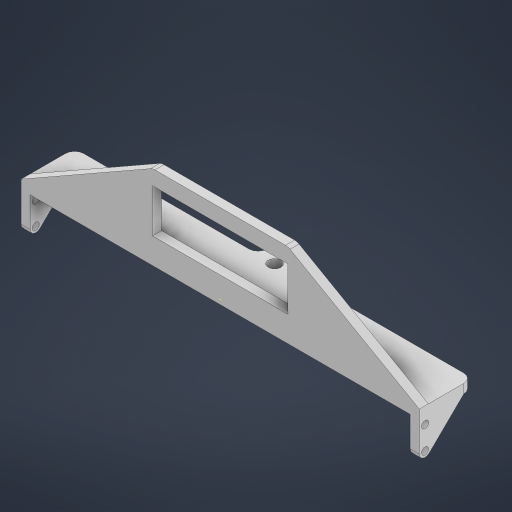
# Autodesk Inventor part: CS_Camera_Mount
Saved by Autodesk Inventor 2023 (Build 270158000, 158)
## iProperties
Created: 2024-02-10
Part Number: CS_Camera_Mount
Material: Generic
Document SubType Name: Modeling
Designer: kelle
Density: 1 g/cm^3
Appearance: Default
Author: kelle
Autodesk Inventor part; units mm, degrees
ref_plane "YZ Plane" through (0, 0, 0) normal (1, 0, 0) x (0, 1, 0)
ref_plane "XZ Plane" through (0, 0, 0) normal (0, 1, 0) x (-1, 0, 0)
ref_plane "XY Plane" through (0, 0, 0) normal (0, 0, 1) x (1, 0, 0)
sketch "Sketch1" plane through (0, 0, 0) normal (0, 0, 1) x (1, 0, 0)
  line L0 (139.7, -3.175) -> (-139.7, -3.175)
  line L1 (-139.7, -3.175) -> (-139.7, 3.175)
  line L2 (-139.7, 3.175) -> (139.7, 3.175)
  line L3 (139.7, 3.175) -> (139.7, -3.175)
  line L4 (139.7, -3.175) -> (-139.7, 3.175) construction
  line L5 (-139.7, -3.175) -> (139.7, 3.175) construction
  point P0 (0, 0)
  dimension "d0" = 279.4
  dimension "d1" = 6.35
  constraints: 12 end point, 2 midpoint, 2 parallel, 1 horizontal, 1 perpendicular
  measures "d0" distance of L1.end L2.end
  measures "d1" distance of L0.end L1.end
extrude "Extrusion1" add sketch "Sketch1" along normal blind 63.5
sketch "Sketch2" plane through (-139.7, 3.175, 0) normal (0, 1, 0) x (1, 0, 0)
  circle A0 centre (140.335, -26) radius 4.445
  line L0 (139.7, 0) -> (139.7, -63.5833) construction
  line L1 (0, 0) -> (0, -63.5) construction
  line L2 (279.4, 0) -> (279.4, -63.5) construction
  line L3 (279.4, -63.5) -> (0, -63.5) projected
  dimension "d4" = 8.89
  dimension "d16" = 37.5
  constraints: 2 end point, 1 centre point, 1 vertical
  measures "d4" diameter of A0
  measures "d16" distance from line of L3 A0.centre
extrude "Extrusion2" cut sketch "Sketch2" against normal through all
sketch "Sketch3" plane through (0, 0, 63.5) normal (0, 0, 1) x (1, 0, 0)
  point P0 (0, 0)
sketch "Sketch4" plane through (-139.7, 3.175, 0) normal (0, 1, 0) x (1, 0, 0)
  line L0 (279.4, 0) -> (279.4, -63.5) projected
  line L1 (0, 0) -> (0, -63.5) projected
  line L2 (279.4, -63.5) -> (0, -63.5)
  line L3 (0, -63.5) -> (0, -57.15)
  line L4 (0, -57.15) -> (279.4, -57.15)
  line L5 (279.4, -57.15) -> (279.4, -63.5)
  point P0 (139.7, 0)
  dimension "d8" = 6.35
  constraints: 8 end point, 2 parallel, 1 horizontal, 1 perpendicular, 1 point on line
  measures "d8" distance of L2.end L3.end
extrude "Extrusion3" add sketch "Sketch4" along normal blind 63.5
sketch "Sketch5" plane through (0, 0, 63.5) normal (0, 0, 1) x (1, 0, 0)
  line L0 (47.5, 14.825) -> (-47.5, 14.825)
  line L1 (-47.5, 14.825) -> (-47.5, 45.305)
  line L2 (-47.5, 45.305) -> (47.5, 45.305)
  line L3 (47.5, 45.305) -> (47.5, 14.825)
  line L4 (47.5, 14.825) -> (-47.5, 45.305) construction
  line L5 (-47.5, 14.825) -> (47.5, 45.305) construction
  line L6 (-139.7, -3.175) -> (139.7, -3.175) projected
  point P0 (0, 0)
  point P1 (0, 30.065)
  dimension "d11" = 95
  dimension "d12" = 30.48
  dimension "d13" = 18
  constraints: 12 end point, 2 midpoint, 2 parallel, 1 horizontal, 1 perpendicular
  measures "d11" distance of L1.end L2.end
  measures "d12" distance of L0.end L1.end
  measures "d13" distance between parallel lines of L6 L0
extrude "Extrusion4" cut sketch "Sketch5" against normal through all
sketch "Sketch8" plane through (0, 0, 63.5) normal (0, 0, 1) x (1, 0, 0)
  line L0 (-139.7, -3.175) -> (139.7, -3.175) construction
  line L1 (-47.5, -3.175) -> (-47.5, 66.9222) construction
  line L2 (-139.7, 66.675) -> (139.7, 66.675) construction
  line L3 (47.5, 66.675) -> (47.5, -3.175) construction
  line L4 (47.5, 45.305) -> (47.5, 14.825) construction
  line L5 (-47.5, 14.825) -> (-47.5, 45.305) construction
  line L6 (-139.7, -3.175) -> (-139.7, 66.675) construction
  line L7 (-139.7, 3.175) -> (139.7, 3.175) construction
  line L8 (139.7, -3.175) -> (139.7, 66.675) construction
  line L9 (-139.7, 55.753) -> (139.7, 55.753)
  line L10 (-47.5, 55.753) -> (-139.7, 3.175)
  line L11 (47.5, 55.753) -> (139.7, 3.175)
  line L12 (-47.5, 14.825) -> (-47.5, 45.305) projected
  line L13 (-47.5, 45.305) -> (47.5, 45.305) projected
  line L14 (47.5, 45.305) -> (47.5, 14.825) projected
  line L15 (47.5, 14.825) -> (-47.5, 14.825) projected
  line L16 (-139.7, -3.175) -> (-139.7, 66.675) projected
  line L17 (-139.7, -3.175) -> (139.7, -3.175) projected
  line L18 (139.7, -3.175) -> (139.7, 66.675) projected
  line L19 (-139.7, 66.675) -> (139.7, 66.675) projected
  point P0 (0, 0)
  point P1 (-47.5, 30.065)
  point P2 (-139.7, 3.175)
  point P3 (139.7, 3.175)
  dimension "d21" = 0
  dimension "d22" = 0
  dimension "d23" = 6.35
  dimension "d24" = 10.922
  constraints: 12 end point, 11 point on line, 2 horizontal, 1 midpoint, 1 perpendicular, 1 vertical
  measures "d21" distance between parallel lines of L4 L3
  measures "d22" distance from line of point (-47.5, 30.065) L1
  measures "d23" distance between parallel lines of L0 L7
  measures "d24" distance between parallel lines of L2 L9
extrude "Extrusion5" cut sketch "Sketch8" against normal through all contours L16 L19 L18 L9 | L9 L10 L16 | L9 L18 L11
sketch "Sketch11" plane through (-139.7, 3.175, 0) normal (0, 1, 0) x (1, 0, 0)
  circle A0 centre (140.335, -26) radius 4.445 projected
  circle A1 centre (140.335, -26) radius 12.7
  line L0 (127.635, -26) -> (0, -26)
  line L1 (0, 0) -> (0, -57.15) projected
  line L2 (153.035, -26) -> (279.4, -26)
  line L3 (279.4, 0) -> (279.4, -57.15) projected
  line L4 (279.4, 0) -> (0, 0) projected
  point P0 (139.7, 0)
  point P1 (0, -34.9602)
  point P2 (280.67, -34.9602)
  point P3 (279.4, -57.15)
  dimension "d43" = 25.4
  constraints: 4 end point, 3 point on line, 2 point on circle, 1 centre point, 1 coincident, 1 horizontal, 2 other
  measures "d43" diameter of A1
extrude "Extrusion8" cut sketch "Sketch11" against normal through all contours A1 L0 L1 L4 L3 L2
fillet "Fillet5" radius 6.35 6 edges at (47.5, 55.753, 60.325) (-47.5, 55.753, 60.325) (139.7, 0, 26) (13.335, 0, 26) (-12.065, 0, 26) (-139.7, 0, 26)
sketch "Sketch15" plane through (-139.7, -3.175, 63.5) normal (-1, 0, 0) x (0, 0, 1)
  circle A0 centre (-4, -5) radius 2.5
  line L0 (-31.15, 0) -> (-31.15, 6.35) projected
  line L1 (-31.15, 0) -> (0, 0) projected
  line L2 (0, 0) -> (0, 6.35) projected
  line L3 (0, 6.35) -> (-6.35, 6.35) projected
  line L4 (-31.15, 6.35) -> (-6.35, 6.35) projected
  line L5 (0, 0) -> (0, -21.002)
  circle A1 centre (-4, -21.002) radius 2.5
  circle A2 centre (-4, -21.002) radius 4
  line L6 (-31.15, 0) -> (0, 0) projected
  line L7 (-31.15, 0) -> (-6.7994, -23.8591)
  point P0 (-63.5, 3.175)
  dimension "d64" = 5
  dimension "d65" = 4
  dimension "d66" = 5
  dimension "d67" = 5
  dimension "d68" = 16.002
  constraints: 4 end point, 3 centre point, 2 point on circle, 2 tangent, 1 coincident, 1 vertical
  measures "d64" diameter of A0
  measures "d65" distance from line of L5 A0.centre
  measures "d66" distance from line of L1 A0.centre
  measures "d67" diameter of A1
  measures "d68" distance of A0.centre A1.centre
extrude "Extrusion11" add sketch "Sketch15" against normal blind 6.35 contours L1 L5 A2 L7 | A2
sketch "Sketch16" plane through (139.7, -3.175, 63.5) normal (1, 0, 0) x (0, 0, -1)
  line L0 (0, 0) -> (0, -21.002) projected
  arc A0 (0, -21.002) -> (6.7994, -23.8591) centre (4, -21.002) ccw projected
  line L1 (6.7994, -23.8591) -> (31.15, 0) projected
  line L2 (0, 0) -> (31.15, 0) projected
  circle A1 centre (4, -5) radius 2.5 projected
  circle A2 centre (4, -21.002) radius 2.5 projected
  point P0 (63.5, 3.175)
extrude "Extrusion12" add sketch "Sketch16" against normal blind 6.35
body "Solid1"
